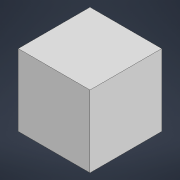
# Autodesk Inventor part: tests1
Saved by Autodesk Inventor 2021 (Build 250183000, 183)
## iProperties
Created: 2021-02-25
Part Number: tests1
Material: Generic
Document SubType Name: Modeling
Designer: lyhol
Density: 1 g/cm^3
Appearance: Default
Author: lyhol
Autodesk Inventor part; units mm, degrees
ref_plane "YZ Plane" through (0, 0, 0) normal (1, 0, 0) x (0, 1, 0)
ref_plane "XZ Plane" through (0, 0, 0) normal (0, 1, 0) x (-1, 0, 0)
ref_plane "XY Plane" through (0, 0, 0) normal (0, 0, 1) x (1, 0, 0)
sketch "Sketch3" plane through (0, 0, 0) normal (1, 0, 0) x (0, 1, 0)
  line L0 (-5, -5) -> (5, -5)
  line L1 (5, -5) -> (5, 5)
  line L2 (5, 5) -> (-5, 5)
  line L3 (-5, 5) -> (-5, -5)
  line L4 (-5, -5) -> (5, 5) construction
  line L5 (5, -5) -> (-5, 5) construction
  point P0 (0, 0)
  dimension "D" = 10
  dimension "B" = 10
  constraints: 12 end point, 2 midpoint, 2 parallel, 1 horizontal, 1 perpendicular
  measures "D" distance of L0.end L1.end
  measures "B" distance of L1.end L2.end
extrude "Extrusion2" add sketch "Sketch3" along normal blind 10
equation "\"B\" = b"
equation "\"d6\" = h_h"
equation "\"b\" = 10"
equation "\"h_h\" = 10"
body "Solid2"
